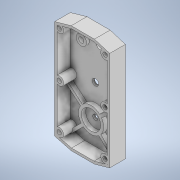
# Autodesk Inventor part: Back half gearbox
Saved by Autodesk Inventor 2020 (Build 240168000, 168)
## iProperties
Created: 2022-05-09
Part Number: Back half gearbox
Material: Generic
Document SubType Name: Modeling
Designer: Administrator
Density: 1 g/cm^3
Appearance: Default
Author: Administrator
Autodesk Inventor part; units mm, degrees
ref_plane "YZ Plane" through (0, 0, 0) normal (1, 0, 0) x (0, 1, 0)
ref_plane "XZ Plane" through (0, 0, 0) normal (0, 1, 0) x (-1, 0, 0)
ref_plane "XY Plane" through (0, 0, 0) normal (0, 0, 1) x (1, 0, 0)
sketch "Sketch1" plane through (0, 0, 0) normal (0, 0, 1) x (1, 0, 0)
  line L0 (-4.445, 2.3537) -> (-11.2171, 2.3537)
  line L1 (-16.0528, 3.6237) -> (-16.0528, 32.5162)
  line L2 (-11.2171, 33.8978) -> (-4.445, 33.8978)
  line L3 (0, 32.5162) -> (0, 3.6237)
  line L4 (-16.0528, 32.5162) -> (-11.2171, 33.8978)
  line L5 (-4.445, 33.8978) -> (0, 32.5162)
  line L6 (-16.0528, 3.6237) -> (-11.2171, 2.3537)
  line L7 (-4.445, 2.3537) -> (0, 3.6237)
  point P0 (0, 0)
  dimension "d13" = 28.8925
  dimension "d14" = 16.0528
  dimension "d15" = 28.8925
  dimension "d16" = 1.27
  dimension "d17" = 4.445
  constraints: 16 end point, 2 parallel, 2 vertical alignment, 1 horizontal, 1 horizontal alignment, 1 perpendicular
  measures "d13" distance of L3.start L3.end
  measures "d14" distance between parallel lines of L3 L1
  measures "d15" distance of L1.start L1.end
  measures "d16" distance from line of L0 L3.end
  measures "d17" distance from line of L3 L0.start
extrude "Extrusion1" add sketch "Sketch1" along normal blind 4.572
shell "Shell1" thickness 0.7112 removed faces 1 at (-8.9597, 23.3831, 4.572)
sketch "Sketch2" plane through (-11.1253, 3.0649, 0.7112) normal (0, 0, 1) x (1, 0, 0)
  circle A0 centre (3.0989, 7.3888) radius 0.762
  line L0 (-0.0918, -0.7112) -> (6.6803, -0.7112) projected
  line L1 (10.4141, 28.9276) -> (10.4141, 1.0953) projected
  line L2 (-4.2163, 1.1073) -> (-4.2163, 28.9148) projected
  circle A1 centre (3.0989, 16.2433) radius 0.9525
  circle A2 centre (9.4743, 20.0769) radius 0.762
  circle A3 centre (4.3435, 26.0069) radius 0.889
  line L3 (11.1253, 0.5588) -> (11.1253, 29.4513) projected
  line L4 (6.6803, -0.7112) -> (11.1253, 0.5588) projected
  line L5 (6.6803, 30.8329) -> (-0.0918, 30.8329) projected
  line L6 (-4.9275, 29.4513) -> (-4.9275, 0.5588) projected
  circle A4 centre (-0.2285, 25.6259) radius 0.762
  circle A5 centre (-0.2285, 25.6259) radius 1.524
  point P0 (11.1253, -3.0649)
  point P1 (3.0989, 15.2908)
  point P2 (10.2363, 20.0769)
  point P3 (9.4743, 19.3149)
  point P4 (9.4743, 0.0871)
  point P5 (4.3435, 26.8959)
  point P6 (3.4545, 26.0069)
  point P7 (-0.2285, 26.3879)
  point P8 (-0.9905, 25.6259)
  dimension "d71" = 1.905
  dimension "d18" = 1.524
  dimension "d19" = 8.1
  dimension "d53" = 7.3152
  dimension "d54" = 14.6304
  dimension "d72" = 16.002
  dimension "d73" = 1.524
  dimension "d74" = 1.778
  dimension "d75" = 0.889
  dimension "d76" = 19.2278
  dimension "d77" = 3.937
  dimension "d78" = 8.382
  dimension "d79" = 1.524
  dimension "d80" = 0.762
  dimension "d81" = 4.445
  dimension "d82" = 3.937
  constraints: 7 vertical alignment, 6 point on circle, 5 centre point, 3 horizontal alignment, 1 point on line, 2 other
  measures "d18" diameter of A0
  measures "d19" distance from line of L0 A0.centre
  measures "d53" distance from line of L1 A0.centre
  measures "d54" distance between parallel lines of L1 L2
  measures "d72" distance from line of L0 point (3.099, 15.291)
  measures "d73" diameter of A2
  measures "d74" diameter of A3
  measures "d75" distance from line of L3 A2.start
  measures "d76" distance of point (9.474, 0.087) A2.end
  measures "d77" distance from line of L5 A3.start
  measures "d78" distance from line of L6 A3.end
  measures "d79" diameter of A4
  measures "d80" radial gap between concentric circles of A4 A5
  measures "d81" distance from line of L5 A4.start
  measures "d82" distance from line of L6 A4.end
extrude "Extrusion2" cut sketch "Sketch2" against normal up to surface (0.7112 mm away) contours A0 | A1 | A2 | A3 | A4
sketch "Sketch3" plane through (-11.1253, 3.0649, 0.7112) normal (0, 0, 1) x (1, 0, 0)
  circle A0 centre (3.0989, 7.3888) radius 0.762 projected
  circle A1 centre (3.0989, 7.3888) radius 2.8194
  circle A2 centre (3.0989, 7.3888) radius 3.6661
  line L0 (6.5806, 0) -> (10.4141, 1.0953) projected
  line L1 (5.3692, 5.7171) -> (10.0851, 1.0013)
  line L2 (5.3745, 4.5145) -> (9.1538, 0.7352)
  line L3 (-4.2163, 1.1073) -> (0, 0) projected
  line L4 (0.8232, 4.5145) -> (-2.9235, 0.7678)
  line L5 (0.8285, 5.7171) -> (-3.8718, 1.0168)
  circle A3 centre (3.0989, 7.3888) radius 0.762 projected
  line L6 (10.4141, 28.9276) -> (10.4141, 1.0953) projected
  line L7 (5.6912, 4.7965) -> (9.6194, 0.8682) construction
  line L8 (0.5066, 4.7965) -> (-3.3976, 0.8923) construction
  line L9 (5.9072, 9.7453) -> (10.4141, 13.527) construction
  line L10 (0.2905, 9.7453) -> (-4.2163, 13.527) construction
  line L11 (-4.2163, 28.9148) -> (-4.2163, 1.1073) projected
  line L12 (5.6163, 10.0538) -> (10.4141, 14.0796)
  line L13 (-4.2163, 12.9744) -> (0.0372, 9.4052)
  line L14 (6.1606, 9.4052) -> (10.4141, 12.9744)
  line L15 (6.5806, 0) -> (0, 0) construction
  line L16 (3.0989, 7.3888) -> (3.0989, 0) construction
  line L17 (3.0989, 7.3888) -> (0.5066, 4.7965) construction
  line L18 (3.0989, 7.3888) -> (5.6912, 4.7965) construction
  line L19 (0.2905, 9.7453) -> (3.0989, 7.3888) construction
  line L20 (5.9072, 9.7453) -> (3.0989, 7.3888) construction
  line L21 (0.5814, 10.0538) -> (-4.2163, 14.0796)
  circle A4 centre (9.7791, 15.2046) radius 0.635
  circle A5 centre (9.7791, 15.2046) radius 1.27
  circle A6 centre (-3.5813, 15.2046) radius 0.635
  circle A7 centre (-3.5813, 15.2046) radius 1.27
  line L22 (-4.2163, 1.1073) -> (-4.2163, 28.9148) projected
  circle A8 centre (-3.5813, 2.2053) radius 0.635
  circle A9 centre (-3.5813, 2.2053) radius 1.27
  circle A10 centre (9.7791, 2.2053) radius 0.635
  circle A11 centre (9.7791, 2.2053) radius 1.27
  circle A12 centre (-3.5813, 28.4359) radius 0.635
  circle A13 centre (-3.5813, 28.4359) radius 1.27
  circle A14 centre (9.7791, 28.46) radius 0.635
  circle A15 centre (9.7791, 28.46) radius 1.27
  line L23 (6.5723, 30.1217) -> (10.4141, 28.9276) projected
  line L24 (-4.2163, 28.9148) -> (0.0078, 30.1217) projected
  point P0 (11.1253, -3.0649)
  point P1 (5.9732, 5.1132)
  point P2 (0.2246, 5.1132)
  point P3 (10.4141, 16.3045)
  point P4 (10.4141, 14.1048)
  point P5 (10.4141, 15.2046)
  point P6 (-4.2163, 16.3045)
  point P7 (-4.2163, 15.2046)
  point P8 (-4.2163, 14.1048)
  point P9 (10.4141, 2.2053)
  point P10 (10.4141, 3.3052)
  point P11 (9.8642, 0.9382)
  point P12 (10.3762, 1.0844)
  point P13 (10.4141, 1.1055)
  point P14 (-3.1323, 1.7563)
  point P15 (-3.5619, 0.9355)
  point P16 (-4.2163, 3.3052)
  point P17 (-4.2163, 2.2053)
  point P18 (9.9675, 29.0664)
  point P19 (8.9172, 29.3928)
  point P20 (10.4141, 27.3602)
  point P21 (10.4141, 28.46)
  point P22 (-2.6983, 29.3486)
  point P23 (-3.7558, 29.0464)
  point P24 (-4.2163, 28.4359)
  point P25 (-4.2163, 27.336)
  dimension "d22" = 5.6388
  dimension "d23" = 0.8467
  dimension "d32" = 85
  dimension "d33" = 85
  dimension "d35" = 0.4233
  dimension "d44" = 45
  dimension "d45" = 0.4233
  dimension "d46" = 0.4233
  dimension "d47" = 0.4233
  dimension "d48" = 0.4233
  dimension "d49" = 45
  dimension "d50" = 0.4233
  dimension "d51" = 0.4233
  dimension "d52" = 0.4233
  dimension "d57" = 1.27
  dimension "d58" = 0.635
  dimension "d59" = 1.27
  dimension "d60" = 0.635
  dimension "d63" = 1.27
  dimension "d64" = 0.635
  dimension "d65" = 1.27
  dimension "d66" = 0.635
  dimension "d67" = 1.27
  dimension "d68" = 0.635
  dimension "d69" = 1.27
  dimension "d70" = 0.635
  constraints: 34 end point, 13 centre point, 13 point on line, 12 tangent, 5 parallel, 4 collinear, 2 point on circle, 1 coincident, 1 vertical, 12 other
  measures "d22" diameter of A1
  measures "d32" angle of L7 L9
  measures "d33" angle of L8 L10
  measures "d35" distance between parallel lines of L10 L13
  measures "d44" angle of L16 L8
  measures "d45" distance between parallel lines of L5 L8
  measures "d46" distance between parallel lines of L8 L4
  measures "d47" distance between parallel lines of L2 L7
  measures "d48" distance between parallel lines of L1 L7
  measures "d49" angle of L16 L7
  measures "d50" distance between parallel lines of L12 L9
  measures "d51" distance between parallel lines of L14 L9
  measures "d52" distance between parallel lines of L10 L21
  measures "d57" diameter of A4
  measures "d58" radial gap between concentric circles of A4 A5
  measures "d59" diameter of A6
  measures "d60" radial gap between concentric circles of A6 A7
  measures "d63" diameter of A8
  measures "d64" radial gap between concentric circles of A8 A9
  measures "d65" diameter of A10
  measures "d66" radial gap between concentric circles of A10 A11
  measures "d67" diameter of A12
  measures "d68" radial gap between concentric circles of A12 A13
  measures "d69" diameter of A14
  measures "d70" radial gap between concentric circles of A14 A15
extrude "Extrusion4" add sketch "Sketch3" along normal blind 1.27 contours A1 L5 A2 L1 | A1 L1 A2 L5 | A2 L4 L3 A9 L5 | L1 A11 L0 L2 A2 | L13 L11 L21 A2 | A9 L3 L5 | L1 L0 A11 | A2 L12 L6 L14
extrude "Extrusion5" add sketch "Sketch3" along normal up to surface (3.8608 mm away) contours A9 L3 L5 | L5 A8 L11 A9 | A11 L6 A10 L1 | L1 L0 A11 | L5 L3 L11 A8 | A10 L6 A11 L0 L1 | L6 A15 L23 A14 | L6 A5 | A12 L24 A13 L11 | A7 L11 picked at (10.1817, 14.2329) picked at (-2.5344, 15.107)
extrude "Extrusion6" add sketch "Sketch2" along normal blind 0.762 contours A5
extrude "Extrusion7" cut sketch "Sketch3" against normal up to surface (0.7112 mm away) contours A8 | A10 | A14 | A4 | A12 | A6
body "Solid1"
